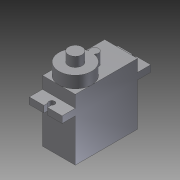
# Autodesk Inventor part: MicroServo_Motor
Saved by Autodesk Inventor 2011 SP2 (Build 150309200, 309)
## iProperties
Created: 2015-10-31
Part Number: MicroServo_Motor
Document SubType Name: Modeling
Designer: Ernest
Density: 1 g/cm^3
Mass: 6.9513 g
Surface Area: 26.3225 cm^2
Volume: 6.9513 cm^3
Author: Ernest
Autodesk Inventor part; units mm, degrees
ref_plane "YZ Plane" through (0, 0, 0) normal (1, 0, 0) x (0, 1, 0)
ref_plane "XZ Plane" through (0, 0, 0) normal (0, 1, 0) x (-1, 0, 0)
ref_plane "XY Plane" through (0, 0, 0) normal (0, 0, 1) x (1, 0, 0)
sketch "Sketch1" plane through (0, 0, 0) normal (0, 0, 1) x (1, 0, 0)
  line L0 (0, 0) -> (-11.375, 0)
  line L1 (-11.375, 0) -> (-11.375, 15.6)
  line L2 (-11.375, 15.6) -> (-16.2, 15.6)
  line L3 (-16.2, 15.6) -> (-16.2, 18)
  line L4 (-16.2, 18) -> (-11.375, 18)
  line L5 (-11.375, 18) -> (-11.375, 22.4)
  line L6 (-11.375, 22.4) -> (11.375, 22.4)
  line L7 (11.375, 22.4) -> (11.375, 18)
  line L8 (11.375, 18) -> (16.2, 18)
  line L9 (16.2, 18) -> (16.2, 15.6)
  line L10 (16.2, 15.6) -> (11.375, 15.6)
  line L11 (11.375, 15.6) -> (11.375, 0)
  line L12 (11.375, 0) -> (0, 0)
  dimension "d0" = 11.375
  dimension "d1" = 15.6
  dimension "d2" = 4.825
  dimension "d3" = 2.4
  dimension "d4" = 4.4
  dimension "d5" = 22.75
  dimension "d7" = 4.825
  dimension "d8" = 2.4
  dimension "d9" = 18
  constraints: 26 end point, 8 perpendicular, 3 parallel, 3 point on line, 1 horizontal
  measures "d0" distance of L0.start L0.end
  measures "d1" distance of L0.end L1.end
  measures "d2" distance of L1.end L2.end
  measures "d3" distance of L2.end L3.end
  measures "d4" distance of L4.end L5.end
  measures "d5" distance of L5.end L6.end
  measures "d7" distance of L7.end L8.end
  measures "d8" distance of L8.end L9.end
  measures "d9" distance between parallel lines of L12 L8
extrude "Extrusion1" add sketch "Sketch1" along normal blind 12
sketch "Sketch2" plane through (-11.375, 22.4, 0) normal (0, 1, 0) x (1, 0, 0)
  line L0 (0, -12) -> (22.75, -12) projected
  line L1 (0, 0) -> (22.75, 0) projected
  line L2 (0, 0) -> (0, -12) projected
  arc A0 (11.9166, -5.003) -> (11.9166, -6.997) centre (6, -6) ccw
  arc A1 (11.9166, -6.997) -> (11.9166, -5.003) centre (13.0373, -6) ccw
  point P0 (11.375, 0)
  dimension "d13" = 3
  constraints: 4 point on circle, 3 tangent, 2 centre point
  measures "d13" diameter of A1
extrude "Extrusion2" add sketch "Sketch2" along normal blind 4.3 contours A0 A1
sketch "Sketch3" plane through (-11.375, 26.7, 0) normal (0, 1, 0) x (1, 0, 0)
  arc A0 (11.9166, -5.003) -> (11.9166, -6.997) centre (6, -6) ccw projected
  circle A1 centre (6, -6) radius 2.5
  point P0 (11.375, 0)
  dimension "d16" = 5
  constraints: 1 centre point, 1 coincident
  measures "d16" diameter of A1
extrude "Extrusion3" add sketch "Sketch3" along normal blind 3.5
sketch "Sketch4" plane through (-16.2, 18, 0) normal (0, 1, 0) x (1, 0, 0)
  line L0 (0, 0) -> (0, -12) projected
  line L1 (27.575, -12) -> (32.4, -12) projected
  line L2 (32.4, 0) -> (32.4, -12) projected
  line L3 (27.575, 0) -> (32.4, 0) projected
  line L4 (27.575, 0) -> (27.575, -12) projected
  arc A0 (1.4254, -6.65) -> (1.4254, -5.35) centre (2.25, -6) ccw
  arc A1 (30.9746, -5.35) -> (30.9746, -6.65) centre (30.15, -6) ccw
  line L5 (0, 0) -> (0, -12) construction
  line L6 (0, -6) -> (32.4, -6) construction
  line L7 (32.4, 0) -> (32.4, -12) construction
  line L8 (0, -5.35) -> (1.4254, -5.35)
  line L9 (0, -6.65) -> (1.4254, -6.65)
  line L10 (32.4, -5.35) -> (30.9746, -5.35)
  line L11 (32.4, -6.65) -> (30.9746, -6.65)
  line L12 (0, -5.35) -> (-0.3532, -5.35)
  line L13 (-0.3532, -5.35) -> (-0.3532, -6.65)
  line L14 (-0.3532, -6.65) -> (0, -6.65)
  line L15 (32.4, -5.35) -> (32.7834, -5.35)
  line L16 (32.7834, -5.35) -> (32.7834, -6.65)
  line L17 (32.7834, -6.65) -> (32.4, -6.65)
  point P0 (16.2, 0)
  dimension "d19" = 2.1
  dimension "d20" = 2.1
  dimension "d21" = 27.9
  dimension "d22" = 2.25
  dimension "d23" = 1.3
  dimension "d25" = 0.65
  dimension "d26" = 1.3
  dimension "d27" = 0.65
  constraints: 22 end point, 6 parallel, 4 point on circle, 4 point on line, 3 perpendicular, 2 centre point, 2 midpoint, 1 collinear
  measures "d19" diameter of A0
  measures "d20" diameter of A1
  measures "d21" distance of A1.centre A0.centre
  measures "d22" distance from line of L0 A0.centre
  measures "d23" distance between parallel lines of L8 L9
  measures "d25" distance between parallel lines of L8 L6
  measures "d26" distance between parallel lines of L11 L10
  measures "d27" distance between parallel lines of L6 L10
extrude "Extrusion4" cut sketch "Sketch4" against normal up to next contours L8 A0 L9 L0 | L0 L14 L13 L12 | L11 A1 L10 L2 | L2 L15 L16 L17
body "Solid1"
